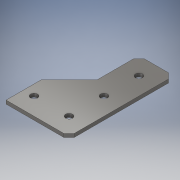
# Autodesk Inventor part: 1in corner bracket for extrusions cut
Saved by Autodesk Inventor 2017 (Build 210142000, 142)
## iProperties
Created: 2016-10-02
Part Number: 1in corner bracket for extrusions cut
Material: Steel, Alloy
Document SubType Name: Modeling
Designer: Aditya
Density: 7.73 g/cm^3
Appearance: Semi-Polished
Author: Aditya
Autodesk Inventor part; units mm, degrees
ref_plane "YZ Plane" through (0, 0, 0) normal (1, 0, 0) x (0, 1, 0)
ref_plane "XZ Plane" through (0, 0, 0) normal (0, 1, 0) x (-1, 0, 0)
ref_plane "XY Plane" through (0, 0, 0) normal (0, 0, 1) x (1, 0, 0)
sketch "Sketch1" plane through (0, 0, 0) normal (0, 1, 0) x (-1, 0, 0)
  line L0 (25.4, -45.72) -> (45.72, -25.4)
  line L1 (0, -3.81) -> (3.81, 0)
  line L2 (3.81, -76.2) -> (0, -72.39)
  line L3 (21.59, -76.2) -> (25.4, -72.39)
  line L4 (0, -3.81) -> (0, -72.39)
  line L5 (3.81, -76.2) -> (21.59, -76.2)
  line L6 (25.4, -72.39) -> (25.4, -45.72)
  circle A0 centre (38.1, -12.7) radius 2.54
  circle A1 centre (12.7, -12.7) radius 2.54
  circle A2 centre (12.7, -38.1) radius 2.54
  circle A3 centre (12.7, -63.5) radius 2.54
  line L7 (45.72, -25.4) -> (45.72, 0)
  line L8 (45.72, 0) -> (3.81, 0)
  point P0 (0, 0)
  constraints: 18 end point, 4 centre point, 3 vertical, 1 horizontal, 1 perpendicular
extrude "Extrusion2" add sketch "Sketch1" along normal blind 2.54
body "Solid2"
